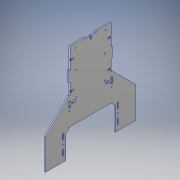
# Autodesk Inventor part: Hopper Wall with Megatronics mount
Saved by Autodesk Inventor 2018 (Build 220112000, 112)
## iProperties
Created: 2013-10-08
Part Number: Hopper Wall with Megatronics mount
Material: Aluminum 6061
Document SubType Name: Modeling
Designer: Gabriel Smolnycki
Mass: 680.384 g
Surface Area: 1344.84 cm^2
Volume: 251.994 cm^3
Density: 2.7 g/cm^3
Appearance: Aluminum - Flat
Sending System: SolidWorks 2017
Last Author: Gabriel Smolnycki
Last Saved: 2017-09-14
Author: Gabriel Smolnycki
Autodesk Inventor part; units mm, degrees
ref_plane "XZ Plane" through (0, 0, 0) normal (0, 1, 0) x (-1, 0, 0)
ref_plane "XY Plane" through (0, 0, 0) normal (0, 0, 1) x (1, 0, 0)
ref_plane "Work Plane1" through (-4, 0, 0) normal (1, 0, 0) x (0, 1, 0)
sketch "Sketch1" plane through (-4, 0, 0) normal (1, 0, 0) x (0, 1, 0)
  arc A0 (-179.834, -64.5065) -> (-185.9063, -63.121) centre (-182, -60) ccw
  line L0 (-264.5, -97.85) -> (-285, -97.85)
  line L1 (-46.75, -63) -> (-46.75, -68)
  line L2 (-146.75, -68) -> (-147.75, -68)
  line L3 (-155.5, 75) -> (-155.5, 79)
  line L4 (-7, 1.75) -> (-7, 2.75)
  line L5 (-285, -97.85) -> (-285, -102.15)
  arc A1 (-191.5, -74.75) -> (-185.9063, -63.121) centre (-191.5, -67.5902) ccw
  line L6 (-195, -74.75) -> (-195, -79.25)
  line L7 (-46.75, -68) -> (-47.75, -68)
  line L8 (-147.75, -68) -> (-147.75, -72)
  line L9 (-46.75, 75) -> (-46.75, 72)
  line L10 (-7, 2.75) -> (-11, 2.75)
  line L11 (-285, 102.15) -> (-285, 97.85)
  line L12 (-195, -79.25) -> (-173.5, -79.25)
  line L13 (-47.75, -68) -> (-47.75, -72)
  line L14 (-147.75, -72) -> (-146.75, -72)
  line L15 (-146.75, 75) -> (-146.75, 72)
  line L16 (-46.75, 72) -> (-47.75, 72)
  line L17 (-11, 2.75) -> (-11, 1.75)
  line L18 (-191.5, -74.75) -> (-195, -74.75)
  line L19 (-143.25, -75) -> (-114.5, -75)
  line L20 (-285, 97.85) -> (-264.5, 97.85)
  line L21 (-173.5, -79.25) -> (-173.5, -74.75)
  line L22 (-47.75, -72) -> (-46.75, -72)
  line L23 (-146.75, -72) -> (-146.75, -75)
  line L24 (-146.75, 72) -> (-147.75, 72)
  line L25 (-47.75, 72) -> (-47.75, 68)
  line L26 (-11, 1.75) -> (-16, 1.75)
  line L27 (-264.5, 97.85) -> (-264.5, 102.15)
  line L28 (-173.5, -74.75) -> (-177.5, -74.75)
  line L29 (-46.75, -72) -> (-46.75, -75)
  line L30 (-155.5, -75) -> (-146.75, -75)
  line L31 (-147.75, 72) -> (-147.75, 68)
  line L32 (-47.75, 68) -> (-46.75, 68)
  line L33 (-16, 1.75) -> (-16, -1.75)
  arc A2 (-179.834, -64.5065) -> (-177.5, -74.75) centre (-177.5, -69.3623) ccw
  line L34 (-75.5, -75) -> (-46.75, -75)
  line L35 (-155.5, -79) -> (-155.5, -75)
  line L36 (-147.75, 68) -> (-146.75, 68)
  line L37 (-46.75, 68) -> (-46.75, 63)
  line L38 (-16, -1.75) -> (-11, -1.75)
  line L39 (-264.5, 102.15) -> (-285, 102.15)
  line L40 (-177.5, 74.75) -> (-173.5, 74.75)
  line L41 (-335, 102.15) -> (-335, 97.85)
  line L42 (-75.5, -79) -> (-75.5, -75)
  line L43 (-241.5, -165) -> (-155.5, -79)
  line L44 (-146.75, 68) -> (-146.75, 63)
  line L45 (-46.75, 63) -> (-43.25, 63)
  line L46 (-11, -1.75) -> (-11, -2.75)
  line L47 (0, 75) -> (-43.25, 75)
  line L48 (-335, 97.85) -> (-314.5, 97.85)
  line L49 (-114.5, -79) -> (-75.5, -79)
  line L50 (-355, -165) -> (-241.5, -165)
  line L51 (-146.75, 63) -> (-143.25, 63)
  line L52 (-43.25, 63) -> (-43.25, 68)
  line L53 (-11, -2.75) -> (-7, -2.75)
  line L54 (-314.5, 97.85) -> (-314.5, 102.15)
  line L55 (-114.5, -75) -> (-114.5, -79)
  line L56 (-355, -90) -> (-355, -165)
  line L57 (-143.25, 63) -> (-143.25, 68)
  line L58 (-43.25, 68) -> (-42.25, 68)
  line L59 (-7, -2.75) -> (-7, -1.75)
  line L60 (0, -75) -> (0, -20)
  line L61 (-270, -90) -> (-355, -90)
  line L62 (-143.25, 68) -> (-142.25, 68)
  line L63 (-42.25, 68) -> (-42.25, 72)
  line L64 (-7, -1.75) -> (-4, -1.75)
  line L65 (-314.5, 102.15) -> (-335, 102.15)
  arc A3 (-177.5, 74.75) -> (-179.834, 64.5065) centre (-177.5, 69.3623) ccw
  line L66 (-43.25, -75) -> (0, -75)
  line L67 (-143.25, -75) -> (-143.25, -72)
  line L68 (-255, -75) -> (-270, -90)
  line L69 (-142.25, 68) -> (-142.25, 72)
  line L70 (-42.25, 72) -> (-43.25, 72)
  line L71 (-4, -1.75) -> (-4, -20)
  arc A4 (-185.9063, 63.121) -> (-191.5, 74.75) centre (-191.5, 67.5902) ccw
  arc A5 (-185.9063, 63.121) -> (-179.834, 64.5065) centre (-182, 60) ccw
  line L72 (-4, -20) -> (0, -20)
  line L73 (-46.75, 75) -> (-75.5, 75)
  line L74 (-314.5, -97.85) -> (-335, -97.85)
  line L75 (-43.25, -75) -> (-43.25, -72)
  line L76 (-143.25, -72) -> (-142.25, -72)
  line L77 (-255, 75) -> (-255, -75)
  line L78 (-142.25, 72) -> (-143.25, 72)
  line L79 (-43.25, 72) -> (-43.25, 75)
  line L80 (-146.75, 75) -> (-155.5, 75)
  line L81 (-335, -97.85) -> (-335, -102.15)
  line L82 (-173.5, 74.75) -> (-173.5, 79.25)
  line L83 (-43.25, -72) -> (-42.25, -72)
  line L84 (-142.25, -72) -> (-142.25, -68)
  line L85 (-270, 90) -> (-255, 75)
  line L86 (-143.25, 72) -> (-143.25, 75)
  line L87 (-335, -102.15) -> (-314.5, -102.15)
  line L88 (-173.5, 79.25) -> (-195, 79.25)
  line L89 (-42.25, -72) -> (-42.25, -68)
  line L90 (-142.25, -68) -> (-143.25, -68)
  line L91 (-355, 90) -> (-270, 90)
  line L92 (-114.5, 75) -> (-143.25, 75)
  line L93 (0, 20) -> (0, 75)
  line L94 (-314.5, -102.15) -> (-314.5, -97.85)
  line L95 (-195, 79.25) -> (-195, 74.75)
  line L96 (-42.25, -68) -> (-43.25, -68)
  line L97 (-143.25, -68) -> (-143.25, -63)
  line L98 (-355, 165) -> (-355, 90)
  line L99 (-114.5, 79) -> (-114.5, 75)
  line L100 (0, 20) -> (-4, 20)
  line L101 (-285, -102.15) -> (-264.5, -102.15)
  line L102 (-195, 74.75) -> (-191.5, 74.75)
  line L103 (-43.25, -68) -> (-43.25, -63)
  line L104 (-143.25, -63) -> (-146.75, -63)
  line L105 (-241.5, 165) -> (-355, 165)
  line L106 (-75.5, 79) -> (-114.5, 79)
  line L107 (-4, 20) -> (-4, 1.75)
  line L108 (-264.5, -102.15) -> (-264.5, -97.85)
  line L109 (-43.25, -63) -> (-46.75, -63)
  line L110 (-146.75, -63) -> (-146.75, -68)
  line L111 (-155.5, 79) -> (-241.5, 165)
  line L112 (-75.5, 75) -> (-75.5, 79)
  line L113 (-4, 1.75) -> (-7, 1.75)
  constraints: 228 end point, 79 equal length, 56 horizontal, 54 vertical, 12 collinear, 12 point on circle, 6 centre point, 2 perpendicular, 1 parallel
extrude "Extrusion5" add sketch "Sketch1" along normal blind 4.064
sketch "Sketch2" plane through (0, 0, 0) normal (1, 0, 0) x (0, 1, 0)
  arc A0 (-174.45, -52.95) -> (-170.95, -52.95) centre (-172.7, -52.95) ccw
  line L0 (-170.95, -52.95) -> (-170.95, -52.45)
  line L1 (-174.45, -52.45) -> (-174.45, -52.95)
  arc A1 (-170.95, -52.45) -> (-174.45, -52.45) centre (-172.7, -52.45) ccw
  constraints: 4 end point, 4 point on circle, 2 centre point, 2 vertical, 1 equal radius, 1 parallel
extrude "Extrusion4" cut sketch "Sketch2" against normal blind 4
sketch "Sketch3" plane through (-4, 0, 0) normal (1, 0, 0) x (0, 1, 0)
  circle A0 centre (-172.7, 52.25) radius 1.75
  constraints: 1 centre point
extrude "Extrusion3" cut sketch "Sketch3" along normal blind 4
sketch "Sketch4" plane through (0, 0, 0) normal (1, 0, 0) x (0, 1, 0)
  line L0 (-88.124, 53.5672) -> (-88.624, 52.8672)
  arc A0 (-88.624, 52.8672) -> (-85.776, 50.8328) centre (-87.2, 51.85) ccw
  line L1 (-85.776, 50.8328) -> (-85.276, 51.5328)
  arc A1 (-85.276, 51.5328) -> (-88.124, 53.5672) centre (-86.7, 52.55) ccw
  constraints: 4 end point, 4 point on circle, 2 centre point, 2 parallel, 1 equal radius
extrude "Extrusion2" cut sketch "Sketch4" against normal blind 4
sketch "Sketch5" plane through (0, 0, 0) normal (1, 0, 0) x (0, 1, 0)
  arc A0 (-88.2652, -53.5326) -> (-85.1348, -51.9674) centre (-86.7, -52.75) ccw
  line L0 (-85.1348, -51.9674) -> (-85.6348, -50.9674)
  line L1 (-88.7652, -52.5326) -> (-88.2652, -53.5326)
  arc A1 (-85.6348, -50.9674) -> (-88.7652, -52.5326) centre (-87.2, -51.75) ccw
  constraints: 4 end point, 4 point on circle, 2 centre point, 2 parallel, 1 equal radius
extrude "Extrusion1" cut sketch "Sketch5" against normal blind 4
hole "Hole6" at (-4, -299.75, -100) direction (1, 0, 0) diameter 3.5 depth 4.064
hole "Hole5" at (-4, -299.75, 100) direction (1, 0, 0) diameter 3.5 depth 4.064
hole "Hole4" at (-4, -205, -77) direction (1, 0, 0) diameter 3.5 depth 4.064
sketch "Sketch8" plane through (-4, 0, 0) normal (1, 0, 0) x (0, 1, 0)
  point P0 (-205, -77)
hole "Hole3" at (-4, -205, 77) direction (1, 0, 0) diameter 3.5 depth 4.064
sketch "Sketch7" plane through (-4, 0, 0) normal (1, 0, 0) x (0, 1, 0)
  point P0 (-299.75, 100)
hole "Hole2" at (-4, -14.5, 55) direction (1, 0, 0) diameter 4.5 depth 4.064
sketch "Sketch6" plane through (-4, 0, 0) normal (1, 0, 0) x (0, 1, 0)
  point P0 (-299.75, -100)
hole "Hole1" at (-4, -14.5, -55) direction (1, 0, 0) diameter 4.5 depth 4.064
sketch "Sketch9" plane through (-4, 0, 0) normal (1, 0, 0) x (0, 1, 0)
  point P0 (-205, 77)
sketch "Sketch10" plane through (-4, 0, 0) normal (1, 0, 0) x (0, 1, 0)
  point P0 (-14.5, 55)
sketch "Sketch11" plane through (-4, 0, 0) normal (1, 0, 0) x (0, 1, 0)
  point P0 (-14.5, -55)
body "Solid3"
